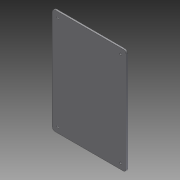
# Autodesk Inventor part: lid
Saved by Autodesk Inventor 2012 (Build 160160000, 160)
## iProperties
Created: 2017-08-16
Part Number: lid
Material: Default
Document SubType Name: Modeling
Designer: Brandon
Density: 1 g/cm^3
Author: Brandon
Autodesk Inventor part; units mm, degrees
ref_plane "YZ Plane" through (0, 0, 0) normal (1, 0, 0) x (0, 1, 0)
ref_plane "XZ Plane" through (0, 0, 0) normal (0, 1, 0) x (-1, 0, 0)
ref_plane "XY Plane" through (0, 0, 0) normal (0, 0, 1) x (1, 0, 0)
sketch "Sketch1" plane through (0, 0, 0) normal (0, 0, 1) x (1, 0, 0)
  line L0 (0, 4.0885) -> (0, 124.7403) projected
  ellipse E0 centre (-3.1759, 124.7385) end of major axis (-0.9296, 126.9848) minor radius 3.175 (0, 124.7403) -> (-3.1741, 127.9144) ccw projected
  line L1 (-3.1741, 127.9144) -> (-35.4736, 127.9144) projected
  line L2 (-53.4736, 127.9144) -> (-85.7259, 127.9144) projected
  ellipse E1 centre (-85.7241, 124.7385) end of major axis (-87.9704, 126.9848) minor radius 3.175 (-85.7259, 127.9144) -> (-88.9, 124.7403) ccw projected
  line L3 (-88.9, 4.0885) -> (-88.9, 124.7403) projected
  ellipse E2 centre (-85.7241, 4.0903) end of major axis (-87.9704, 1.844) minor radius 3.175 (-88.9, 4.0885) -> (-85.7259, 0.9144) ccw projected
  line L4 (-85.7259, 0.9144) -> (-61.8967, 0.9144) projected
  line L5 (-30.7967, 0.9144) -> (-3.1741, 0.9144) projected
  ellipse E3 centre (-3.1759, 4.0903) end of major axis (-0.9296, 1.844) minor radius 3.175 (-3.1741, 0.9144) -> (0, 4.0885) ccw projected
  circle A0 centre (-6.5913, 7.5057) radius 1.1938 projected
  circle A1 centre (-13.8176, 14.732) radius 1.1938 projected
  circle A2 centre (-82.3087, 7.5057) radius 1.1938 projected
  circle A3 centre (-75.0824, 14.732) radius 1.1938 projected
  circle A4 centre (-82.3087, 121.3231) radius 1.1938 projected
  circle A5 centre (-75.0824, 114.0968) radius 1.1938 projected
  circle A6 centre (-6.5913, 121.3231) radius 1.1938 projected
  circle A7 centre (-13.8176, 114.0968) radius 1.1938 projected
  line L6 (-53.4736, 127.9144) -> (-35.4736, 127.9144)
  line L7 (-61.8967, 0.9144) -> (-30.7967, 0.9144)
  point P0 (0, 0)
  constraints: 4 end point, 1 collinear, 1 parallel, 4 other
extrude "Extrusion1" add sketch "Sketch1" along normal blind 2.0066 contours E3 L5 L7 L4 E2 L3 E1 L2 L6 L1 E0 L0 | A1 | A3 | A5 | A7
chamfer "Chamfer1" distance 2.0066 distance2 2.0066 1 edges at (-7.7851, 121.3231, 2.0066) measured on face at (-48.7223, 43.2477, 2.0066)
chamfer "Chamfer2" distance 2.0066 distance2 2.0066 1 edges at (-83.5025, 121.3231, 2.0066) measured on face at (-48.7223, 43.2477, 2.0066)
chamfer "Chamfer3" distance 2.0066 distance2 2.0066 1 edges at (-83.5025, 7.5057, 2.0066) measured on face at (-48.7223, 43.2477, 2.0066)
chamfer "Chamfer4" distance 2.0066 distance2 2.0066 1 edges at (-7.7851, 7.5057, 2.0066) measured on face at (-54.9204, 46.3227, 2.0066)
body "Solid1"
